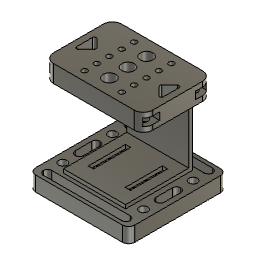
Double NEMA 17 Motor Mount v7 (Autodesk Fusion 360 design; units mm, degrees)
Autodesk Fusion 360 part; units mm, degrees
sketch "Sketch1" plane through (0, 0, 0) normal (0, 0, 1) x (1, 0, 0) in component "Motor Mounts (Constraints)"
  line L0 (25, -27) -> (-25, -27)
  line L1 (-25, -27) -> (-25, 27)
  line L2 (-25, 27) -> (25, 27)
  line L3 (25, 27) -> (25, -27)
  line L4 (-12.85, -15) -> (-12.85, 15)
  line L5 (12.85, 15) -> (12.85, -15)
  line L6 (-17, 15) -> (-17, -15)
  line L7 (17, -15) -> (17, 15)
  line L8 (12.85, 15) -> (17, 15)
  line L9 (17, -15) -> (12.85, -15)
  line L10 (-12.85, -15) -> (-17, -15)
  line L11 (-17, 15) -> (-12.85, 15)
  line L12 (-14.925, 0) -> (-14.925, -10)
  line L13 (-14.925, 0) -> (-14.925, 10)
  line L14 (15, 0) -> (15, 10)
  line L15 (15, 0) -> (15, -10)
  line L16 (-25, 27) -> (25, 27)
  line L17 (25, 27) -> (25, 24)
  line L18 (25, 24) -> (-25, 24)
  line L19 (-25, 24) -> (-25, 27)
  dimension "d1" = 50
  dimension "d2" = 54
  dimension "d7" = 3
  constraint horizontal L0
  constraint perpendicular L0 L1
  constraint parallel L0 L2
  constraint parallel L1 L3
  constraint parallel L4 L5
  constraint parallel L6 L7
  constraint perpendicular L5 L8
  constraint perpendicular L5 L9
  constraint perpendicular L6 L10
  constraint perpendicular L4 L11
  constraint perpendicular L11 L12
  constraint parallel L12 L13
  constraint vertical L14
  constraint parallel L14 L15
  constraint horizontal L16
  constraint vertical L17
  constraint horizontal L18
  constraint vertical L19
  measures "d1" distance of L1.end L2.end
  measures "d2" distance of L0.end L1.end
  measures "d7" distance of L1.end L18.end
extrude "Extrude1" add sketch "Sketch1" along normal blind 3 contours L0 L1 L3 L18 makes body 1 in component "Motor Mounts (Constraints)"
extrude "Extrude2" add sketch "Sketch1" along normal blind 52 contours L1 L2 L3 L16 L17 L18 L19 bodies 1 in component "Motor Mounts (Constraints)"
sketch "Base" plane through (0, 0, 0) normal (0, 0, 1) x (1, 0, 0) in component "Base Piece"
  line L0 (15, -10) -> (-15, 10) construction
  line L1 (-15, -10) -> (15, 10) construction
  line L2 (25, -27) -> (-25, -27)
  line L3 (-25, -27) -> (-25, 27)
  line L4 (-25, 27) -> (25, 27)
  line L5 (25, 27) -> (25, -27)
  circle A0 centre (15, 10) radius 2.125
  circle A1 centre (15, -10) radius 2.125
  circle A2 centre (-15, -10) radius 2.125
  circle A3 centre (-15, 10) radius 2.125
  line L6 (-12.9793, 6.5) -> (-10.9585, 10)
  line L7 (-10.9585, 10) -> (-12.9793, 13.5)
  line L8 (-12.9793, 13.5) -> (-17.0207, 13.5)
  line L9 (-17.0207, 13.5) -> (-19.0415, 10)
  line L10 (-19.0415, 10) -> (-17.0207, 6.5)
  line L11 (-17.0207, 6.5) -> (-12.9793, 6.5)
  line L12 (-12.9793, -13.5) -> (-10.9585, -10)
  line L13 (-10.9585, -10) -> (-12.9793, -6.5)
  line L14 (-12.9793, -6.5) -> (-17.0207, -6.5)
  line L15 (-17.0207, -6.5) -> (-19.0415, -10)
  line L16 (-19.0415, -10) -> (-17.0207, -13.5)
  line L17 (-17.0207, -13.5) -> (-12.9793, -13.5)
  line L18 (17.0207, 6.5) -> (19.0415, 10)
  line L19 (19.0415, 10) -> (17.0207, 13.5)
  line L20 (17.0207, 13.5) -> (12.9793, 13.5)
  line L21 (12.9793, 13.5) -> (10.9585, 10)
  line L22 (10.9585, 10) -> (12.9793, 6.5)
  line L23 (12.9793, 6.5) -> (17.0207, 6.5)
  line L24 (12.9793, -6.5) -> (10.9585, -10)
  line L25 (10.9585, -10) -> (12.9793, -13.5)
  line L26 (12.9793, -13.5) -> (17.0207, -13.5)
  line L27 (17.0207, -13.5) -> (19.0415, -10)
  line L28 (19.0415, -10) -> (17.0207, -6.5)
  line L29 (17.0207, -6.5) -> (12.9793, -6.5)
  circle A4 centre (-15, 20) radius 2.125
  circle A5 centre (15, 20) radius 2.125
  circle A6 centre (15, 0) radius 2.125
  circle A7 centre (-15, 0) radius 2.125
  line L30 (-12.9793, 16.5) -> (-10.9585, 20)
  line L31 (-10.9585, 20) -> (-12.9793, 23.5)
  line L32 (-12.9793, 23.5) -> (-17.0207, 23.5)
  line L33 (-17.0207, 23.5) -> (-19.0415, 20)
  line L34 (-19.0415, 20) -> (-17.0207, 16.5)
  line L35 (-17.0207, 16.5) -> (-12.9793, 16.5)
  line L36 (-12.9793, -3.5) -> (-10.9585, 0)
  line L37 (-10.9585, 0) -> (-12.9793, 3.5)
  line L38 (-12.9793, 3.5) -> (-17.0207, 3.5)
  line L39 (-17.0207, 3.5) -> (-19.0415, 0)
  line L40 (-19.0415, 0) -> (-17.0207, -3.5)
  line L41 (-17.0207, -3.5) -> (-12.9793, -3.5)
  line L42 (17.0207, 16.5) -> (19.0415, 20)
  line L43 (19.0415, 20) -> (17.0207, 23.5)
  line L44 (17.0207, 23.5) -> (12.9793, 23.5)
  line L45 (12.9793, 23.5) -> (10.9585, 20)
  line L46 (10.9585, 20) -> (12.9793, 16.5)
  line L47 (12.9793, 16.5) -> (17.0207, 16.5)
  line L48 (12.9793, 3.5) -> (10.9585, 0)
  line L49 (10.9585, 0) -> (12.9793, -3.5)
  line L50 (12.9793, -3.5) -> (17.0207, -3.5)
  line L51 (17.0207, -3.5) -> (19.0415, 0)
  line L52 (19.0415, 0) -> (17.0207, 3.5)
  line L53 (17.0207, 3.5) -> (12.9793, 3.5)
  circle A8 centre (-32.5, 20) radius 7.5
  circle A9 centre (-32.5, 20) radius 5
  circle A10 centre (-32.5, 20) radius 3.375
  circle A11 centre (32.5, 20) radius 3.375
  circle A12 centre (32.5, 20) radius 7.5
  circle A13 centre (32.5, 20) radius 5
  circle A14 centre (-32.5, -20) radius 3.375
  circle A15 centre (-32.5, -20) radius 7.5
  circle A16 centre (-32.5, -20) radius 5
  circle A17 centre (32.5, -20) radius 3.375
  circle A18 centre (32.5, -20) radius 7.5
  circle A19 centre (32.5, -20) radius 5
  line L54 (35, -39.5) -> (-35, -39.5)
  line L55 (-40, -34.5) -> (-40, 34.5)
  line L56 (-35, 39.5) -> (35, 39.5)
  line L57 (40, 34.5) -> (40, -34.5)
  line L58 (-35, 33.125) -> (-35, 33.375)
  line L59 (35, 33.375) -> (35, 33.125)
  line L60 (-35, -33.375) -> (-35, -33.125)
  line L61 (35, -33.125) -> (35, -33.375)
  circle A20 centre (-15, -20) radius 2.125
  circle A21 centre (15, -20) radius 2.125
  line L62 (-17.0207, -16.5) -> (-19.0415, -20)
  line L63 (-19.0415, -20) -> (-17.0207, -23.5)
  line L64 (-17.0207, -23.5) -> (-12.9793, -23.5)
  line L65 (-12.9793, -23.5) -> (-10.9585, -20)
  line L66 (-10.9585, -20) -> (-12.9793, -16.5)
  line L67 (-12.9793, -16.5) -> (-17.0207, -16.5)
  line L68 (12.9793, -16.5) -> (10.9585, -20)
  line L69 (10.9585, -20) -> (12.9793, -23.5)
  line L70 (12.9793, -23.5) -> (17.0207, -23.5)
  line L71 (17.0207, -23.5) -> (19.0415, -20)
  line L72 (19.0415, -20) -> (17.0207, -16.5)
  line L73 (17.0207, -16.5) -> (12.9793, -16.5)
  arc A22 (-35, 39.5) -> (-40, 34.5) centre (-35, 34.5) ccw
  arc A23 (40, 34.5) -> (35, 39.5) centre (35, 34.5) ccw
  arc A24 (35, -39.5) -> (40, -34.5) centre (35, -34.5) ccw
  arc A25 (-40, -34.5) -> (-35, -39.5) centre (-35, -34.5) ccw
  line L74 (40, -27.5) -> (-40, -27.5)
  line L75 (-40, 27.5) -> (40, 27.5)
  line L76 (-29.2668, 14.4) -> (-26.0337, 20)
  line L77 (-26.0337, 20) -> (-29.2668, 25.6)
  line L78 (-29.2668, 25.6) -> (-35.7332, 25.6)
  line L79 (-35.7332, 14.4) -> (-29.2668, 14.4)
  line L80 (-35.7332, 25.6) -> (-40, 25.6)
  line L81 (-35.7332, 14.4) -> (-40, 14.4)
  line L82 (35.7332, 25.6) -> (29.2668, 25.6)
  line L83 (29.2668, 25.6) -> (26.0337, 20)
  line L84 (26.0337, 20) -> (29.2668, 14.4)
  line L85 (29.2668, 14.4) -> (35.7332, 14.4)
  line L86 (35.7332, 14.4) -> (40, 14.4)
  line L87 (35.7332, 25.6) -> (40, 25.6)
  line L88 (-29.2668, -25.6) -> (-26.0337, -20)
  line L89 (-26.0337, -20) -> (-29.2668, -14.4)
  line L90 (-29.2668, -14.4) -> (-35.7332, -14.4)
  line L91 (-35.7332, -25.6) -> (-29.2668, -25.6)
  line L92 (-35.7332, -25.6) -> (-40, -25.6)
  line L93 (-35.7332, -14.4) -> (-40, -14.4)
  line L94 (35.7332, -14.4) -> (29.2668, -14.4)
  line L95 (29.2668, -14.4) -> (26.0337, -20)
  line L96 (26.0337, -20) -> (29.2668, -25.6)
  line L97 (29.2668, -25.6) -> (35.7332, -25.6)
  line L98 (35.7332, -14.4) -> (40, -14.4)
  line L99 (35.7332, -25.6) -> (40, -25.6)
  line L100 (31.675, 36.625) -> (-31.675, 36.625)
  line L101 (-35, 33.3) -> (-35, 33.2)
  line L102 (-31.675, 29.875) -> (31.675, 29.875)
  line L103 (35, 33.2) -> (35, 33.3)
  line L104 (31.675, -36.625) -> (-31.675, -36.625)
  line L105 (-35, -33.3) -> (-35, -33.2)
  line L106 (-31.675, -29.875) -> (31.675, -29.875)
  line L107 (35, -33.2) -> (35, -33.3)
  arc A26 (-31.675, 36.625) -> (-35, 33.3) centre (-31.675, 33.3) ccw
  arc A27 (-35, 33.2) -> (-31.675, 29.875) centre (-31.675, 33.2) ccw
  arc A28 (31.675, 29.875) -> (35, 33.2) centre (31.675, 33.2) ccw
  arc A29 (35, 33.3) -> (31.675, 36.625) centre (31.675, 33.3) ccw
  arc A30 (-35, -33.3) -> (-31.675, -36.625) centre (-31.675, -33.3) ccw
  arc A31 (-31.675, -29.875) -> (-35, -33.2) centre (-31.675, -33.2) ccw
  arc A32 (35, -33.2) -> (31.675, -29.875) centre (31.675, -33.2) ccw
  arc A33 (31.675, -36.625) -> (35, -33.3) centre (31.675, -33.3) ccw
  line L108 (-32.45, 10) -> (-32.55, 10)
  line L109 (-35.875, 6.675) -> (-35.875, -6.675)
  line L110 (-32.55, -10) -> (-32.45, -10)
  line L111 (-29.125, -6.675) -> (-29.125, 6.675)
  line L112 (32.55, -10) -> (32.45, -10)
  line L113 (29.125, -6.675) -> (29.125, 6.675)
  line L114 (32.45, 10) -> (32.55, 10)
  line L115 (35.875, 6.675) -> (35.875, -6.675)
  arc A34 (-32.55, 10) -> (-35.875, 6.675) centre (-32.55, 6.675) ccw
  arc A35 (-29.125, 6.675) -> (-32.45, 10) centre (-32.45, 6.675) ccw
  arc A36 (-32.45, -10) -> (-29.125, -6.675) centre (-32.45, -6.675) ccw
  arc A37 (-35.875, -6.675) -> (-32.55, -10) centre (-32.55, -6.675) ccw
  arc A38 (32.45, 10) -> (29.125, 6.675) centre (32.45, 6.675) ccw
  arc A39 (35.875, 6.675) -> (32.55, 10) centre (32.55, 6.675) ccw
  arc A40 (29.125, -6.675) -> (32.45, -10) centre (32.45, -6.675) ccw
  arc A41 (32.55, -10) -> (35.875, -6.675) centre (32.55, -6.675) ccw
  circle A42 centre (0, -20) radius 5
  circle A43 centre (0, 20) radius 5
  line L116 (0.01, -10) -> (-0.01, -10)
  line L117 (-5, -5.01) -> (-5, 5.01)
  line L118 (-0.01, 10) -> (0.01, 10)
  line L119 (5, 5.01) -> (5, -5.01)
  arc A44 (-0.01, 10) -> (-5, 5.01) centre (-0.01, 5.01) ccw
  arc A45 (5, 5.01) -> (0.01, 10) centre (0.01, 5.01) ccw
  arc A46 (0.01, -10) -> (5, -5.01) centre (0.01, -5.01) ccw
  arc A47 (-5, -5.01) -> (-0.01, -10) centre (-0.01, -5.01) ccw
  point P0 (-15, 10)
  point P1 (-15, -10)
  point P2 (15, 10)
  point P3 (15, -10)
  point P4 (-15, 20)
  point P5 (-15, 0)
  point P6 (15, 20)
  point P7 (15, 0)
  point P8 (0, 33.25)
  point P9 (0, -33.25)
  point P10 (-35, 31.125)
  point P11 (-35, 35.375)
  point P12 (0, 33.25)
  point P13 (-35, -35.375)
  point P14 (-35, -31.125)
  point P15 (0, -33.25)
  point P16 (-15, -20)
  point P17 (15, -20)
  point P18 (-32.5, 20)
  point P19 (32.5, 20)
  point P20 (-32.5, -20)
  point P21 (32.5, -20)
  point P22 (-35, 29.875)
  point P23 (35, 29.875)
  point P24 (0, 33.25)
  point P25 (0, -33.25)
  point P26 (-35.875, 10)
  point P27 (-35.875, -10)
  point P28 (-29.125, -10)
  point P29 (-32.5, 0)
  point P30 (32.5, 0)
  dimension "d14" = 4.25
  dimension "d15" = 4.25
  dimension "d16" = 4.25
  dimension "d17" = 4.25
  dimension "d18" = 3.5
  dimension "d19" = 3.5
  dimension "d20" = 3.5
  dimension "d21" = 3.5
  dimension "d22" = 4.25
  dimension "d23" = 4.25
  dimension "d24" = 4.25
  dimension "d25" = 4.25
  dimension "d26" = 3.5
  dimension "d27" = 3.5
  dimension "d28" = 3.5
  dimension "d29" = 3.5
  dimension "d36" = 10
  dimension "d37" = 6.75
  dimension "d44" = 4.25
  dimension "d45" = 4.25
  dimension "d46" = 3.5
  dimension "d47" = 3.5
  dimension "d48" = 5
  dimension "d61" = 5.6
  dimension "d62" = 5.6
  dimension "d63" = 5.6
  dimension "d64" = 5.6
  dimension "d87" = 3.325
  dimension "d88" = 6.75
  dimension "d89" = 20
  dimension "d92" = 3.325
  dimension "d93" = 10
  dimension "d96" = 4.99
  constraint coincident L0 origin
  constraint coincident L1 origin
  constraint horizontal L2
  constraint perpendicular L2 L3
  constraint parallel L2 L4
  constraint parallel L3 L5
  constraint coincident P2 L1.end
  constraint coincident P3 L0.start
  constraint coincident P1 L1.start
  constraint coincident P0 L0.end
  constraint coincident P4 A4.centre
  constraint coincident P5 A7.centre
  constraint coincident P6 A5.centre
  constraint coincident P7 A6.centre
  constraint concentric A8 A9
  constraint concentric A8 A10
  constraint horizontal L54
  constraint perpendicular L54 L55
  constraint parallel L54 L56
  constraint parallel L55 L57
  constraint coincident P24 P12
  constraint coincident P25 P15
  constraint coincident P16 A20.centre
  constraint coincident P17 A21.centre
  constraint tangent L55 A22
  constraint tangent L56 A22
  constraint tangent L56 A23
  constraint tangent L57 A23
  constraint equal A22 A23
  constraint tangent L54 A24
  constraint tangent L57 A24
  constraint equal A22 A24
  constraint tangent L54 A25
  constraint tangent L55 A25
  constraint equal A22 A25
  constraint coincident P11 L58
  constraint coincident P10 L58
  constraint coincident P13 L60
  constraint coincident P14 L60
  constraint horizontal L74
  constraint parallel L74 L75
  constraint coincident P18 A8.centre
  constraint coincident L55 L80.end
  constraint perpendicular L55 L80
  constraint coincident L55 L81.end
  constraint perpendicular L55 L81
  constraint coincident P19 A11.centre
  constraint coincident L57 L86.end
  constraint perpendicular L57 L86
  constraint coincident L57 L87.end
  constraint perpendicular L57 L87
  constraint coincident P20 A14.centre
  constraint coincident L55 L92.end
  constraint perpendicular L55 L92
  constraint coincident L55 L93.end
  constraint perpendicular L55 L93
  constraint coincident P21 A17.centre
  constraint coincident L57 L98.end
  constraint perpendicular L57 L98
  constraint coincident L57 L99.end
  constraint perpendicular L57 L99
  constraint horizontal L100
  constraint horizontal L104
  constraint tangent L100 A26
  constraint tangent L101 A26
  constraint coincident P22 L101
  constraint coincident P22 L102
  constraint tangent L101 A27
  constraint tangent L102 A27
  constraint equal A26 A27
  constraint coincident P23 L102
  constraint coincident P23 L103
  constraint tangent L102 A28
  constraint tangent L103 A28
  constraint equal A26 A28
  constraint tangent L100 A29
  constraint tangent L103 A29
  constraint equal A26 A29
  constraint tangent L104 A30
  constraint tangent L105 A30
  constraint equal A26 A30
  constraint tangent L105 A31
  constraint tangent L106 A31
  constraint equal A26 A31
  constraint tangent L106 A32
  constraint tangent L107 A32
  constraint equal A26 A32
  constraint tangent L104 A33
  constraint tangent L107 A33
  constraint equal A26 A33
  constraint horizontal L108
  constraint perpendicular L108 L109
  constraint parallel L108 L110
  constraint parallel L109 L111
  constraint horizontal L112
  constraint perpendicular L112 L113
  constraint parallel L112 L114
  constraint parallel L113 L115
  constraint coincident P26 L108
  constraint coincident P26 L109
  constraint tangent L108 A34
  constraint tangent L109 A34
  constraint tangent L108 A35
  constraint tangent L111 A35
  constraint equal A34 A35
  constraint coincident P28 L110
  constraint coincident P28 L111
  constraint tangent L110 A36
  constraint tangent L111 A36
  constraint equal A34 A36
  constraint coincident P27 L109
  constraint coincident P27 L110
  constraint tangent L109 A37
  constraint tangent L110 A37
  constraint equal A34 A37
  constraint tangent L113 A38
  constraint tangent L114 A38
  constraint equal A34 A38
  constraint tangent L114 A39
  constraint tangent L115 A39
  constraint equal A34 A39
  constraint tangent L112 A40
  constraint tangent L113 A40
  constraint equal A34 A40
  constraint tangent L112 A41
  constraint tangent L115 A41
  constraint equal A34 A41
  constraint horizontal L116
  constraint perpendicular L116 L117
  constraint parallel L116 L118
  constraint parallel L117 L119
  constraint tangent L117 A44
  constraint tangent L118 A44
  constraint tangent L118 A45
  constraint tangent L119 A45
  constraint equal A44 A45
  constraint tangent L116 A46
  constraint tangent L119 A46
  constraint equal A44 A46
  constraint tangent L116 A47
  constraint tangent L117 A47
  constraint equal A44 A47
  measures "d14" diameter of A0
  measures "d15" diameter of A1
  measures "d16" diameter of A2
  measures "d17" diameter of A3
  measures "d18" distance of P0 L11
  measures "d19" distance of P1 L17
  measures "d20" distance of P2 L23
  measures "d21" distance of P3 L29
  measures "d22" diameter of A4
  measures "d23" diameter of A5
  measures "d24" diameter of A6
  measures "d25" diameter of A7
  measures "d26" distance of P4 L35
  measures "d27" distance of P5 L41
  measures "d28" distance of P6 L47
  measures "d29" distance of P7 L53
  measures "d36" diameter of A9
  measures "d37" diameter of A10
  measures "d44" diameter of A20
  measures "d45" diameter of A21
  measures "d46" distance of P16 L67
  measures "d47" distance of P17 L73
  measures "d48" radius of A22
  measures "d61" distance of P18 L79
  measures "d62" distance of P19 L85
  measures "d63" distance of P20 L91
  measures "d64" distance of P21 L97
  measures "d87" radius of A26
  measures "d88" distance of P27 P28
  measures "d89" distance of P26 P27
  measures "d92" radius of A34
  measures "d93" diameter of A42
  measures "d96" radius of A44
extrude "Extrude1'" add sketch "Base" along normal blind 12 separate body contours L2 L3 L5 A15 A18 L74 | L2 L3 L4 L5 | L5 A12 A18 L57 L86 L98 | A18 L94 L95 L96 L97 L98 L99 | L3 A8 A15 L55 L81 L93 | A15 L88 L89 L90 L91 L92 L93 | L3 L4 L5 A8 A12 L75 | A12 L82 L83 L84 L85 L86 L87 | A18 L57 L98 | A18 L94 L95 L96 L97 L98 L99 | A18 L57 L74 L99 | L54 L55 L57 A24 A25 L74 | A8 L76 L77 L78 L79 L80 L81 | A15 L88 L89 L90 L91 L92 L93 | A15 L55 L93 | A15 L55 L74 L92 | A12 L57 L75 L87 | L55 L56 L57 A22 A23 L75 | A12 L82 L83 L84 L85 L86 L87 | A12 L57 L86 | A18 L57 L99 | A8 L55 L75 L80 | A8 L55 L81 | A8 L76 L77 L78 L79 L80 L81 | A15 L55 L92 | A12 L57 L87 | A8 L55 L80 makes body 2 in component "Base Piece"
extrude "Extrude2'" add sketch "Base" along normal blind 7 from surface at 5 contours L6 L7 L8 L9 L10 L11 | L12 L13 L14 L15 L16 L17 | L18 L19 L20 L21 L22 L23 | L24 L25 L26 L27 L28 L29 | L30 L31 L32 L33 L34 L35 | L36 L37 L38 L39 L40 L41 | L42 L43 L44 L45 L46 L47 | L48 L49 L50 L51 L52 L53 | L62 L63 L64 L65 L66 L67 | L68 L69 L70 L71 L72 L73 bodies 2 in component "Base Piece"
extrude "Extrude3" add sketch "Base" along normal up to surface (5 mm away) from surface at 7 contours A9 | A13 | A16 | A19 bodies 2 in component "Base Piece"
sketch "Sketch2" plane through (0, 0, 0) normal (1, 0, 0) x (0, 1, 0) in component "Base Piece"
  line L0 (0, 6) -> (20, 6)
  line L1 (0, 6) -> (-20, 6)
extrude "Extrude4" add sketch "Base" along normal blind 4 separate body contours L2 L3 L5 A15 A18 L74 | L2 L3 L4 L5 | L5 A12 A18 L57 L86 L98 | A18 L94 L95 L96 L97 L98 L99 | L3 A8 A15 L55 L81 L93 | A15 L88 L89 L90 L91 L92 L93 | L3 L4 L5 A8 A12 L75 | A12 L82 L83 L84 L85 L86 L87 | A18 L57 L98 | A18 L94 L95 L96 L97 L98 L99 | A8 L76 L77 L78 L79 L80 L81 | A15 L88 L89 L90 L91 L92 L93 | A15 L55 L93 | A12 L82 L83 L84 L85 L86 L87 | A12 L57 L86 | A8 L55 L81 | A8 L76 L77 L78 L79 L80 L81 | A9 | A13 | A16 | A19 | L108 L109 L110 L111 A34 A35 A36 A37 | L112 L113 L114 L115 A38 A39 A40 A41 | A42 | A43 | L116 L117 L118 L119 A44 A45 A46 A47 makes body 3 in component "Base Piece"
extrude "Extrude5" add sketch "Base" along normal blind 9 contours L2 L3 L5 A15 A18 L74 | L2 L3 L4 L5 | L5 A12 A18 L57 L86 L98 | A18 L94 L95 L96 L97 L98 L99 | L3 A8 A15 L55 L81 L93 | A15 L88 L89 L90 L91 L92 L93 | L3 L4 L5 A8 A12 L75 | A12 L82 L83 L84 L85 L86 L87 | A8 L76 L77 L78 L79 L80 L81 | L108 L109 L110 L111 A34 A35 A36 A37 | L112 L113 L114 L115 A38 A39 A40 A41 | A42 | A43 | L116 L117 L118 L119 A44 A45 A46 A47 picked at (32.5, -26.2333) picked at (-32.5, -26.2333) picked at (32.5, 26.2333) picked at (-32.5, 26.2333) bodies 3 in component "Base Piece"
extrude "Extrude6" add sketch "Base" along normal blind 2 from surface at 9 contours L2 L3 L5 A15 A18 L74 | L2 L3 L4 L5 | L5 A12 A18 L57 L86 L98 | A18 L94 L95 L96 L97 L98 L99 | L3 A8 A15 L55 L81 L93 | A15 L88 L89 L90 L91 L92 L93 | L3 L4 L5 A8 A12 L75 | A12 L82 L83 L84 L85 L86 L87 | A18 L57 L98 | A18 L94 L95 L96 L97 L98 L99 | A8 L76 L77 L78 L79 L80 L81 | A15 L88 L89 L90 L91 L92 L93 | A15 L55 L93 | A12 L82 L83 L84 L85 L86 L87 | A12 L57 L86 | A8 L55 L81 | A8 L76 L77 L78 L79 L80 L81 | L6 L7 L8 L9 L10 L11 | L12 L13 L14 L15 L16 L17 | L18 L19 L20 L21 L22 L23 | L24 L25 L26 L27 L28 L29 | L30 L31 L32 L33 L34 L35 | L36 L37 L38 L39 L40 L41 | L42 L43 L44 L45 L46 L47 | L48 L49 L50 L51 L52 L53 | A9 | A13 | A16 | A19 | L62 L63 L64 L65 L66 L67 | L68 L69 L70 L71 L72 L73 | L108 L109 L110 L111 A34 A35 A36 A37 | L112 L113 L114 L115 A38 A39 A40 A41 | A42 | A43 | L116 L117 L118 L119 A44 A45 A46 A47 bodies 3 in component "Base Piece"
extrude "Extrude7" add sketch "Base" along normal blind 2 from surface at 11 contours L2 L3 L5 A15 A18 L74 | L2 L3 L4 L5 | L5 A12 A18 L57 L86 L98 | A18 L94 L95 L96 L97 L98 L99 | L3 A8 A15 L55 L81 L93 | A15 L88 L89 L90 L91 L92 L93 | L3 L4 L5 A8 A12 L75 | A12 L82 L83 L84 L85 L86 L87 | A18 L57 L98 | A18 L94 L95 L96 L97 L98 L99 | A8 L76 L77 L78 L79 L80 L81 | A15 L88 L89 L90 L91 L92 L93 | A15 L55 L93 | A12 L82 L83 L84 L85 L86 L87 | A12 L57 L86 | A8 L55 L81 | A8 L76 L77 L78 L79 L80 L81 | L6 L7 L8 L9 L10 L11 | L12 L13 L14 L15 L16 L17 | L18 L19 L20 L21 L22 L23 | L24 L25 L26 L27 L28 L29 | L30 L31 L32 L33 L34 L35 | L36 L37 L38 L39 L40 L41 | L42 L43 L44 L45 L46 L47 | L48 L49 L50 L51 L52 L53 | A9 | A10 | A11 | A13 | A14 | A16 | A17 | A19 | L62 L63 L64 L65 L66 L67 | L68 L69 L70 L71 L72 L73 | L108 L109 L110 L111 A34 A35 A36 A37 | L112 L113 L114 L115 A38 A39 A40 A41 | A42 | A43 | L116 L117 L118 L119 A44 A45 A46 A47 bodies 3 in component "Base Piece"
move_body "Move1" bodies 3 to x (1, 0, 0) y (0, 1, 0) z (0, 0, 1) at (0, 0, 60) in component "Base Piece"
move_body "Move1'" bodies 1 to x (1, 0, 0) y (0, 1, 0) z (0, 0, 1) at (0, 0, 12) in component "Motor Mounts (Constraints)"
move_body "Move2" bodies 3 to x (1, 0, 0) y (0, 1, 0) z (0, 0, 1) at (0, 0, 11) in component "Base Piece"
extrude "Extrude10" cut 4 faces at (38.5136, 17.6452, 80) (38.5136, -17.6452, 80) (-38.5136, -17.6452, 80) (-38.5136, 17.6452, 80) along direction (0, 0, 1) blind 1 on bodies 3 bodies 3 in component "Base Piece"
extrude "Extrude9" cut 4 faces at (31.449, -19.348, 82) (-33.208, -21.9396, 82) (-33.208, 18.0604, 82) (31.449, 20.652, 82) along direction (0, 0, 1) blind 1 on bodies 3 bodies 3 in component "Base Piece"
extrude "Extrude11" add 1 faces at (-32.375, 0, 84) along direction (0, 0, 1) blind 1 on bodies 3 bodies 3 in component "Base Piece"
sketch "Cutouts" plane through (0, 0, 0) normal (0, 0, 1) x (1, 0, 0) in component "Base Piece"
  circle A0 centre (0, 15) radius 5
  circle A1 centre (0, -15) radius 5
  line L0 (23.99, -7.5) -> (24.01, -7.5)
  line L1 (26, -9.49) -> (26, -15.51)
  line L2 (24.01, -17.5) -> (23.99, -17.5)
  line L3 (22, -15.51) -> (22, -9.49)
  arc A2 (23.99, -7.5) -> (22, -9.49) centre (23.99, -9.49) ccw
  arc A3 (26, -9.49) -> (24.01, -7.5) centre (24.01, -9.49) ccw
  arc A4 (24.01, -17.5) -> (26, -15.51) centre (24.01, -15.51) ccw
  arc A5 (22, -15.51) -> (23.99, -17.5) centre (23.99, -15.51) ccw
  circle A6 centre (23, 0) radius 2
  circle A7 centre (-23.9998, -0.0958) radius 2
  circle A8 centre (0, 0) radius 5
  line L4 (-24.01, -7.5) -> (-23.99, -7.5)
  line L5 (-22, -9.49) -> (-22, -15.51)
  arc A9 (-24.01, -7.5) -> (-26, -9.49) centre (-24.01, -9.49) ccw
  line L6 (-23.99, -17.5) -> (-24.01, -17.5)
  arc A10 (-22, -9.49) -> (-23.99, -7.5) centre (-23.99, -9.49) ccw
  line L7 (-26, -15.51) -> (-26, -9.49)
  arc A11 (-23.99, -17.5) -> (-22, -15.51) centre (-23.99, -15.51) ccw
  arc A12 (-26, -15.51) -> (-24.01, -17.5) centre (-24.01, -15.51) ccw
  line L8 (23.99, 17.5) -> (24.01, 17.5)
  line L9 (26, 15.51) -> (26, 9.49)
  arc A13 (23.99, 17.5) -> (22, 15.51) centre (23.99, 15.51) ccw
  line L10 (24.01, 7.5) -> (23.99, 7.5)
  arc A14 (26, 15.51) -> (24.01, 17.5) centre (24.01, 15.51) ccw
  line L11 (22, 9.49) -> (22, 15.51)
  arc A15 (24.01, 7.5) -> (26, 9.49) centre (24.01, 9.49) ccw
  arc A16 (22, 9.49) -> (23.99, 7.5) centre (23.99, 9.49) ccw
  line L12 (-24.01, 17.5) -> (-23.99, 17.5)
  line L13 (-22, 15.51) -> (-22, 9.49)
  arc A17 (-24.01, 17.5) -> (-26, 15.51) centre (-24.01, 15.51) ccw
  line L14 (-23.99, 7.5) -> (-24.01, 7.5)
  arc A18 (-22, 15.51) -> (-23.99, 17.5) centre (-23.99, 15.51) ccw
  line L15 (-26, 9.49) -> (-26, 15.51)
  arc A19 (-23.99, 7.5) -> (-22, 9.49) centre (-23.99, 9.49) ccw
  arc A20 (-26, 9.49) -> (-24.01, 7.5) centre (-24.01, 9.49) ccw
  line L16 (35, 0) -> (35, 6.3787)
  line L17 (35, 0) -> (35, -6.3787)
  line L18 (26.0607, 1.0607) -> (32.4393, 7.4393)
  line L19 (32.4393, -7.4393) -> (26.0607, -1.0607)
  arc A21 (32.4393, -7.4393) -> (35, -6.3787) centre (33.5, -6.3787) ccw
  arc A22 (26.0607, 1.0607) -> (26.0607, -1.0607) centre (27.1213, 0) ccw
  arc A23 (35, 6.3787) -> (32.4393, 7.4393) centre (33.5, 6.3787) ccw
  line L20 (0, 0) -> (0, 3)
  arc A24 (-35, -6.3787) -> (-32.4393, -7.4393) centre (-33.5, -6.3787) ccw
  line L21 (-35, 0) -> (-35, -6.3787)
  line L22 (-32.4393, -7.4393) -> (-26.0607, -1.0607)
  arc A25 (-32.4393, 7.4393) -> (-35, 6.3787) centre (-33.5, 6.3787) ccw
  line L23 (-26.0607, 1.0607) -> (-32.4393, 7.4393)
  line L24 (-35, 0) -> (-35, 6.3787)
  arc A26 (-26.0607, -1.0607) -> (-26.0607, 1.0607) centre (-27.1213, 0) ccw
  point P0 (24, -15)
  point P1 (-24, -15)
  point P2 (24, 10)
  point P3 (-24, 10)
  dimension "d105" = -48
  dimension "d106" = 25
  dimension "d109" = 1.5
  constraint tangent L0 A2
  constraint tangent L3 A2
  constraint tangent L0 A3
  constraint tangent L1 A3
  constraint tangent L1 A4
  constraint tangent L2 A4
  constraint tangent L2 A5
  constraint tangent L3 A5
  constraint coincident A8.centre L20.start
  constraint vertical L16
  constraint parallel L16 L17
  constraint perpendicular L18 L19
  constraint tangent L17 A21
  constraint tangent L19 A21
  constraint tangent L18 A22
  constraint tangent L19 A22
  constraint equal A21 A22
  constraint tangent L16 A23
  constraint tangent L18 A23
  constraint equal A21 A23
  constraint vertical L20
  constraint symmetric L16.start L20 L21.start
  constraint symmetric L17.end L20 A24.start
  constraint symmetric L19.start L20 A24.end
  constraint symmetric A21 L20 A24
  constraint symmetric L18.start L20 L23.start
  constraint symmetric L19.end L20 L22.end
  constraint symmetric A22 L20 A26
  constraint symmetric L16.end L20 A25.end
  constraint symmetric L18.end L20 A25.start
  constraint symmetric A23 L20 A25
  measures "d109" radius of A21
extrude "Extrude14" cut sketch "Cutouts" along normal blind 100 contours A7 A26 | A7 A24 L21 L22 A25 L23 L24 A26 | L16 L17 L18 L19 A21 A22 A23 picked at (-25.8672, 0.1185) bodies 3 in component "Base Piece"
extrude "Extrude13" cut sketch "Cutouts" along normal blind 100 contours A0 | A1 | A8 bodies 3 in component "Base Piece"
component "Motor Mounts (Constraints)" placed x (1, 0, 0) y (0, 1, 0) z (0, 0, 1) at (0, 0, 0)
component "Base Piece" placed x (1, 0, 0) y (0, 1, 0) z (0, 0, 1) at (0, 0, 0)
component "Base Piece" placed x (1, 0, 0) y (0, 1, 0) z (0, 0, 1) at (0, 0, 0)
named bodies: "PE Motor Constraints", "PE Dual Motor Mount Bottom Base", "PE Dual Motor Mount Top Base"
